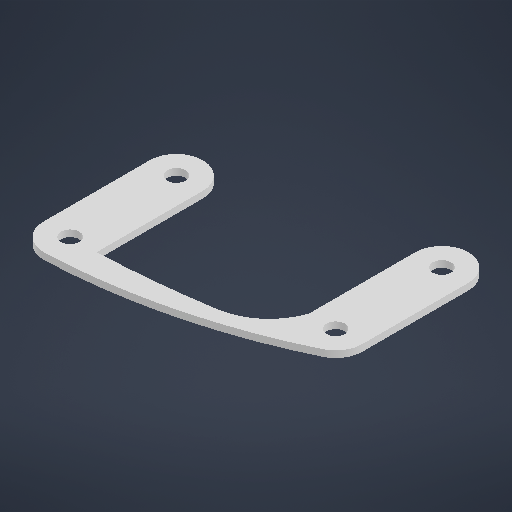
# Autodesk Inventor part: backfunnel
Saved by Autodesk Inventor 2025.2 (Build 292293000, 293)
## iProperties
Created: 2025-03-22
Part Number: backfunnel
Material: Generic
Document SubType Name: Modeling
Designer: Jahan
Density: 1 g/cm^3
Appearance: Default
Author: Jahan
Autodesk Inventor part; units mm, degrees
ref_plane "YZ Plane" through (0, 0, 0) normal (1, 0, 0) x (0, 1, 0)
ref_plane "XZ Plane" through (0, 0, 0) normal (0, 1, 0) x (-1, 0, 0)
ref_plane "XY Plane" through (0, 0, 0) normal (0, 0, 1) x (1, 0, 0)
sketch "Sketch1" plane through (0, 0, 0) normal (0, 1, 0) x (-1, 0, 0)
  circle A0 centre (35.1094, 28.5187) radius 2.1844
  circle A1 centre (35.1094, 3.1187) radius 2.1844
  circle A2 centre (-15.6906, 15.8187) radius 2.1844
  circle A3 centre (-15.6906, -9.5813) radius 2.1844
  circle A4 centre (35.1094, 28.5187) radius 6.35
  circle A5 centre (35.1094, 3.1187) radius 6.35
  circle A6 centre (-15.6906, 15.8187) radius 6.35
  circle A7 centre (-15.6906, -9.5813) radius 6.35
  line L0 (-22.0406, -9.5813) -> (-22.0406, 15.8187)
  line L1 (-9.3406, -9.5813) -> (-9.3406, 15.8187)
  line L2 (28.7594, 3.1187) -> (28.7594, 28.5187)
  line L3 (41.4594, 28.5187) -> (41.4594, 3.1187)
  arc A8 (28.7594, 28.5187) -> (-15.6906, 22.1687) centre (37.4719, -191.2191) ccw
  arc A9 (34.8585, 34.8637) -> (-18.4551, 21.5353) centre (40.1808, -99.7171) ccw
  arc A10 (2.5131, 25.8949) -> (-9.3406, 15.8187) centre (4.8989, 11.0777) ccw
  point P0 (0, 0)
  point P1 (-9.3406, 15.8187)
  point P2 (28.7594, 28.5187)
  dimension "d0" = 12.7
  dimension "d1" = 12.7
  dimension "d2" = 12.7
  dimension "d3" = 12.7
  constraints: 20 point on circle, 11 centre point, 9 tangent, 8 end point, 4 coincident, 1 vertical
  measures "d0" diameter of A4
  measures "d1" diameter of A5
  measures "d2" diameter of A6
  measures "d3" diameter of A7
extrude "Extrusion1" add sketch "Sketch1" along normal blind 1.5875
body "Solid1"
